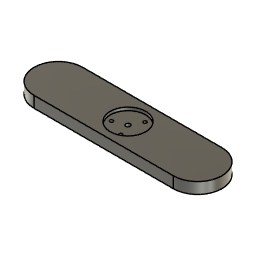
부품1 v2 (Autodesk Fusion 360 design; units mm, degrees)
Autodesk Fusion 360 part; units mm, degrees
sketch "스케치1" plane through (0, 0, 0) normal (0, 0, 1) x (1, 0, 0)
  line L0 (0, 0) -> (116, 0)
  line L1 (116, 0) -> (116, 30)
  line L2 (116, 30) -> (0, 30)
  line L3 (0, 30) -> (0, 0)
  dimension "d1" = 116
  dimension "d2" = 30
  constraint horizontal L0
  constraint vertical L1
  constraint horizontal L2
  constraint vertical L3
  constraint coincident L0.start L3.end
  measures "d1" distance of L0.start L0.end
  measures "d2" distance of L0.start L2.end
extrude "돌출1" add sketch "스케치1" along normal blind 5
fillet "필렛1" radius 15 4 edges at (0, 0, 2.5) (116, 0, 2.5) (116, 30, 2.5) (0, 30, 2.5)
sketch "스케치2" plane through (0, 0, 5) normal (0, 0, 1) x (-1, 0, 0)
  arc A0 (-15, -30) -> (-15, 0) centre (-15, -15) ccw
  line L0 (-15, 0) -> (-101, 0)
  arc A1 (-101, 0) -> (-101, -30) centre (-101, -15) ccw
  line L1 (-101, -30) -> (-15, -30)
  circle A2 centre (-58, -15) radius 10.95
  dimension "d7" = 15
  dimension "d8" = 58
  dimension "d9" = 21.9
  measures "d7" distance of L1 A2.centre
  measures "d8" horizontal distance of origin A2.centre
  measures "d9" diameter of A2
extrude "돌출2" add sketch "스케치2" along normal blind 1.9
sketch "스케치3" plane through (0, 0, 5) normal (0, 0, 1) x (-1, 0, 0)
  circle A0 centre (-58, -15) radius 10.95
  circle A1 centre (-58, -15) radius 1.4
  circle A2 centre (-58, -15) radius 7.8085 construction
  circle A3 centre (-61.6659, -21.8945) radius 1
  circle A4 centre (-50.7199, -12.1763) radius 1
  circle A5 centre (-60.8237, -7.7199) radius 1
  line L0 (-61.6659, -21.8945) -> (-58, -15) construction
  line L1 (-58, -15) -> (-50.7199, -12.1763) construction
  line L2 (-58, -15) -> (-60.8237, -7.7199) construction
  line L3 (-58, -15) -> (-58, -25.95) construction
  dimension "d12" = 2.8
  dimension "d13" = 15.617
  dimension "d14" = 2
  dimension "d15" = 2
  dimension "d16" = 2
  dimension "d17" = 90
  dimension "d18" = 139.2
  dimension "d20" = 28
  constraint concentric A0 A1
  constraint concentric A1 A2
  constraint coincident A2 A3.centre
  constraint coincident A2 A4.centre
  constraint coincident A2 A5.centre
  constraint coincident A3.centre L0.start
  constraint coincident A0.centre A1.centre
  constraint coincident A4.centre L1.end
  constraint coincident A5.centre L2.end
  constraint coincident A0 L3.end
  constraint vertical L3
  measures "d12" diameter of A1
  measures "d13" diameter of A2
  measures "d14" diameter of A3
  measures "d15" diameter of A4
  measures "d16" diameter of A5
  measures "d17" angle of L1 L2
  measures "d18" angle of L0 L1
  measures "d20" angle of L0 L3
extrude "돌출3" cut sketch "스케치3" against normal blind 5 contours A1 | A3 | A4 | A5
equation "d8 = ( 116 / 2 ) * 1 mm"
